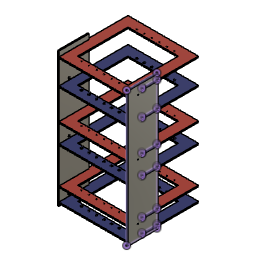
ionenantrieb v1 v3 (Autodesk Fusion 360 design; units mm, degrees)
Autodesk Fusion 360 part; units mm, degrees
sketch "Skizze1" plane through (0, 0, 0) normal (0, 0, 1) x (1, 0, 0)
  line L0 (0, 0) -> (100, 0)
  line L1 (100, 0) -> (100, 100)
  line L2 (100, 100) -> (0, 100)
  line L3 (0, 100) -> (0, 0)
  line L4 (-17.4, -20) -> (120, -20)
  line L5 (120, -20) -> (120, 120)
  line L6 (120, 120) -> (-20, 120)
  line L7 (-20, 120) -> (-20, 10)
  line L8 (-20, 10) -> (-17.4, 10)
  line L9 (-17.4, 10) -> (-17.4, -20)
  line L10 (50, 0) -> (50, 5)
  line L11 (117.4, 10) -> (117.4, -20)
  line L12 (120, 10) -> (117.4, 10)
  dimension "d1" = 100
  dimension "d2" = 100
  dimension "d4" = 2.6
  dimension "d5" = 30
  constraint horizontal L0
  constraint vertical L1
  constraint horizontal L2
  constraint vertical L3
  constraint coincident L0.start L3.end
  constraint perpendicular L7 L8
  constraint perpendicular L4 L9
  constraint parallel L0 L4
  constraint parallel L1 L5
  constraint parallel L2 L6
  constraint parallel L3 L7
  constraint midpoint L0 L10.start
  constraint perpendicular L0 L10
  constraint symmetric L7.end L10 L12.start
  constraint symmetric L8.end L10 L11.start
  constraint symmetric L4.start L10 L11.end
  measures "d1" distance of L1.end L2.end
  measures "d2" distance of L0.start L2.end
  measures "d4" distance of L7.end L8.end
  measures "d5" distance of L8.end L4.start
extrude "Extrusion1" add sketch "Skizze1" along normal blind 2.5 contours L4 L5 L6 L7 L8 L9 L11 L12 makes body 1
sketch "Skizze2" plane through (-17.4, 0, 0) normal (-1, 0, 0) x (0, -1, 0)
  line L0 (20, -5) -> (20, 117.8288)
  line L1 (-10, 0) -> (20, 0)
  line L2 (20, -5) -> (-40, -5)
  line L3 (-40, -5) -> (-40, -0.05)
  line L4 (-40, -0.05) -> (-10, -0.05)
  line L5 (-10, -0.05) -> (-10, 2.55)
  line L6 (-10, 2.55) -> (-40, 2.55)
  line L7 (-40, 2.55) -> (-40, 27.55)
  line L8 (-40, 15.05) -> (-27, 15.05)
  line L9 (-40, 30.15) -> (-10, 30.15)
  line L10 (-10, 30.15) -> (-10, 27.55)
  line L11 (-10, 27.55) -> (-40, 27.55)
  line L12 (-40, 30.15) -> (-40, 99.95)
  line L13 (-40, 102.55) -> (-10, 102.55)
  line L14 (-10, 102.55) -> (-10, 99.95)
  line L15 (-10, 199.95) -> (-40, 199.95)
  line L16 (-10, 202.55) -> (-10, 199.95)
  line L17 (-40, 202.55) -> (-10, 202.55)
  line L18 (-10, 138.4115) -> (-40, 138.4115)
  line L19 (-10, 141.0115) -> (-10, 138.4115)
  line L20 (-40, 141.0115) -> (-10, 141.0115)
  line L21 (-10, 249.95) -> (-40, 249.95)
  line L22 (-40, 252.55) -> (-10, 252.55)
  line L23 (-10, 252.55) -> (-10, 249.95)
  line L24 (-40, 252.55) -> (-40, 262.55)
  line L25 (-40, 262.55) -> (20, 262.55)
  line L26 (20, 262.55) -> (20, 117.8288)
  line L27 (-40, 249.95) -> (-40, 202.55)
  line L28 (-40, 199.95) -> (-40, 141.0115)
  line L29 (-40, 138.4115) -> (-40, 102.55)
  line L30 (-40, 99.95) -> (-10, 99.95)
  dimension "d37" = 5
  dimension "d38" = 4.95
  dimension "d39" = 2.6
  dimension "d40" = 25
  dimension "d41" = 100
  dimension "d42" = 10
  dimension "d43" = 60
  dimension "d44" = 60
  dimension "d45" = 60
  dimension "d46" = 60
  dimension "d47" = 60
  dimension "d49" = 60
  constraint vertical L0
  constraint perpendicular L0 L2
  constraint perpendicular L2 L3
  constraint perpendicular L3 L4
  constraint perpendicular L1 L5
  constraint perpendicular L5 L6
  constraint perpendicular L6 L7
  constraint midpoint L7 L8.start
  constraint perpendicular L7 L8
  constraint symmetric L3.end L8 L9.start
  constraint symmetric L4.end L8 L9.end
  constraint symmetric L5.end L8 L10.end
  constraint symmetric L6.end L8 L7.end
  constraint perpendicular L9 L12
  constraint perpendicular L22 L24
  constraint perpendicular L24 L25
  constraint perpendicular L17 L27
  constraint perpendicular L20 L28
  constraint perpendicular L13 L29
  constraint perpendicular L14 L30
  measures "d37" distance of L0.start L1
  measures "d38" distance of L2.end L3.end
  measures "d39" distance of L4.end L5.end
  measures "d40" distance of L6.end L7.end
  measures "d41" distance of L3.end L12.end
  measures "d42" distance of L22.start L24.end
  measures "d43" distance of L0.start L2.end
  measures "d44" distance of L0 L7
  measures "d45" distance of L0.end L29
  measures "d46" distance of L26 L28
  measures "d47" distance of L26 L27
  measures "d49" distance of L24 L26
extrude "Extrusion2" add sketch "Skizze2" along normal blind 2.5 separate body makes body 2
ref_plane "Arbeitsebene1" through (-18.65, 25, 15.05) normal (0, 0, 1) x (0, 1, 0)
mirror "Spiegeln1" about plane through (-18.65, 25, 15.05) normal (0, 0, 1) of bodies 1 makes body 3
ref_plane "Arbeitsebene2" through (50, 65, 28.85) normal (1, 0, 0) x (0, 1, 0)
mirror "Spiegeln2" about plane through (50, 65, 28.85) normal (1, 0, 0) of bodies 2 makes body 4
sketch "Skizze3" plane through (0, 0, 2.5) normal (0, 0, 1) x (-1, 0, 0)
  line L0 (0, 0) -> (0, -100)
  line L1 (0, -100) -> (-100, -100)
  line L2 (-100, -100) -> (-100, 0)
  line L3 (-100, 0) -> (0, 0)
  line L4 (-120, -120) -> (20, -120)
  line L5 (20, -120) -> (20, -10)
  line L6 (20, -10) -> (17.4, -10)
  line L7 (17.4, -10) -> (17.4, 20)
  line L8 (17.4, 20) -> (-117.4, 20)
  line L9 (-117.4, 20) -> (-117.4, -10)
  line L10 (-117.4, -10) -> (-120, -10)
  line L11 (-120, -10) -> (-120, -120)
  circle A0 centre (-12.5, -105) radius 2
  circle A1 centre (-27.5, -105) radius 2
  circle A2 centre (-42.5, -105) radius 2
  circle A3 centre (-57.5, -105) radius 2
  circle A4 centre (-72.5, -105) radius 2
  line L12 (0, -50) -> (-0.7928, -50)
  circle A5 centre (-27.5, 5) radius 2
  circle A6 centre (-72.5, 5) radius 2
  circle A7 centre (-42.5, 5) radius 2
  circle A8 centre (-57.5, 5) radius 2
  circle A9 centre (-12.5, 5) radius 2
  circle A10 centre (-87.5, -105) radius 2
  circle A11 centre (-87.5, 5) radius 2
  point P0 (-87.5, 5)
  dimension "d16" = 4
  dimension "d17" = 5
  dimension "d18" = 12.5
  dimension "d21" = 75
  dimension "d22" = 0
  constraint midpoint L0 L12.start
  constraint perpendicular L0 L12
  constraint symmetric A0 L12 A9
  constraint symmetric A1 L12 A5
  constraint symmetric A2 L12 A7
  constraint symmetric A3 L12 A8
  constraint symmetric A4 L12 A6
  constraint symmetric L12 A10.centre P0
  constraint symmetric L12 A10 A11
  measures "d16" diameter of A0
  measures "d17" distance of L1 A0.centre
  measures "d18" distance of L0 A0.centre
extrude "Extrusion3" cut sketch "Skizze3" against normal blind 2.5 contours A0 | A1 | A2 | A3 | A4 | A5 | A6 | A7 | A8 | A9 | A10 | A11 bodies 1
sketch "Skizze4" plane through (0, 0, 30.1) normal (0, 0, 1) x (-1, 0, 0)
  line L0 (0, 0) -> (0, -100)
  line L1 (0, -100) -> (-100, -100)
  line L2 (-100, -100) -> (-100, 0)
  line L3 (-100, 0) -> (0, 0)
  line L4 (-120, -120) -> (20, -120)
  line L5 (20, -120) -> (20, -10)
  line L6 (20, -10) -> (17.4, -10)
  line L7 (17.4, -10) -> (17.4, 20)
  line L8 (17.4, 20) -> (-117.4, 20)
  line L9 (-117.4, 20) -> (-117.4, -10)
  line L10 (-117.4, -10) -> (-120, -10)
  line L11 (-120, -10) -> (-120, -120)
  circle A0 centre (-12.5, -105) radius 1
  circle A1 centre (-27.5, -105) radius 1
  circle A2 centre (-42.5, -105) radius 1
  circle A3 centre (-57.5, -105) radius 1
  circle A4 centre (-72.5, -105) radius 1
  line L12 (0, -50) -> (-0.625, -50)
  circle A5 centre (-27.5, 5) radius 1
  circle A6 centre (-72.5, 5) radius 1
  circle A7 centre (-42.5, 5) radius 1
  circle A8 centre (-12.5, 5) radius 1
  circle A9 centre (-57.5, 5) radius 1
  circle A10 centre (-87.5, -105) radius 1
  circle A11 centre (-87.5, 5) radius 1
  dimension "d25" = 2
  dimension "d26" = 5
  dimension "d27" = 12.5
  dimension "d30" = 75
  dimension "d31" = 0
  constraint midpoint L0 L12.start
  constraint perpendicular L0 L12
  constraint symmetric A0 L12 A8
  constraint symmetric A1 L12 A5
  constraint symmetric A2 L12 A7
  constraint symmetric A3 L12 A9
  constraint symmetric A4 L12 A6
  constraint symmetric L12 A10 A11
  measures "d25" diameter of A0
  measures "d26" distance of L1 A0.centre
  measures "d27" distance of L0 A0.centre
extrude "Extrusion4" cut sketch "Skizze4" against normal blind 2.5 contours A0 | A1 | A2 | A3 | A4 | A5 | A6 | A7 | A8 | A9 | A10 | A11 bodies 3
sketch "Skizze5" plane through (117.4, 0, 0) normal (-1, 0, 0) x (0, -1, 0)
  line L0 (-40, 30.15) -> (-10, 30.15)
  line L1 (-10, 30.15) -> (-10, 27.55)
  line L2 (-10, 27.55) -> (-40, 27.55)
  line L3 (-40, 27.55) -> (-40, 2.55)
  line L4 (-40, 2.55) -> (-10, 2.55)
  line L5 (-10, 2.55) -> (-10, -0.05)
  line L6 (-10, -0.05) -> (-40, -0.05)
  line L7 (-40, -0.05) -> (-40, -5)
  line L8 (-40, -5) -> (20, -5)
  line L9 (20, -5) -> (20, 262.55)
  line L10 (20, 262.55) -> (-40, 262.55)
  line L11 (-40, 262.55) -> (-40, 252.55)
  line L12 (-40, 252.55) -> (-10, 252.55)
  line L13 (-10, 252.55) -> (-10, 249.95)
  line L14 (-10, 249.95) -> (-40, 249.95)
  line L15 (-40, 249.95) -> (-40, 202.55)
  line L16 (-40, 202.55) -> (-10, 202.55)
  line L17 (-10, 202.55) -> (-10, 199.95)
  line L18 (-10, 199.95) -> (-40, 199.95)
  line L19 (-40, 199.95) -> (-40, 141.0115)
  line L20 (-40, 141.0115) -> (-10, 141.0115)
  line L21 (-10, 141.0115) -> (-10, 138.4115)
  line L22 (-10, 138.4115) -> (-40, 138.4115)
  line L23 (-40, 138.4115) -> (-40, 102.55)
  line L24 (-40, 102.55) -> (-10, 102.55)
  line L25 (-10, 102.55) -> (-10, 99.95)
  line L26 (-10, 99.95) -> (-40, 99.95)
  line L27 (-40, 99.95) -> (-40, 30.15)
sketch "Skizze6" plane through (-19.9, 0, 0) normal (-1, 0, 0) x (0, -1, 0)
  line L0 (-40, 30.15) -> (-10, 30.15)
  line L1 (-10, 30.15) -> (-10, 27.55)
  line L2 (-10, 27.55) -> (-40, 27.55)
  line L3 (-40, 27.55) -> (-40, 2.55)
  line L4 (-40, 2.55) -> (-10, 2.55)
  line L5 (-10, 2.55) -> (-10, -0.05)
  line L6 (-10, -0.05) -> (-40, -0.05)
  line L7 (-40, -0.05) -> (-40, -5)
  line L8 (-40, -5) -> (20, -5)
  line L9 (20, -5) -> (20, 262.55)
  line L10 (20, 262.55) -> (-40, 262.55)
  line L11 (-40, 262.55) -> (-40, 252.55)
  line L12 (-40, 252.55) -> (-10, 252.55)
  line L13 (-10, 252.55) -> (-10, 249.95)
  line L14 (-10, 249.95) -> (-40, 249.95)
  line L15 (-40, 249.95) -> (-40, 202.55)
  line L16 (-40, 202.55) -> (-10, 202.55)
  line L17 (-10, 202.55) -> (-10, 199.95)
  line L18 (-10, 199.95) -> (-40, 199.95)
  line L19 (-40, 199.95) -> (-40, 141.0115)
  line L20 (-40, 141.0115) -> (-10, 141.0115)
  line L21 (-10, 141.0115) -> (-10, 138.4115)
  line L22 (-10, 138.4115) -> (-40, 138.4115)
  line L23 (-40, 138.4115) -> (-40, 102.55)
  line L24 (-40, 102.55) -> (-10, 102.55)
  line L25 (-10, 102.55) -> (-10, 99.95)
  line L26 (-10, 99.95) -> (-40, 99.95)
  line L27 (-40, 99.95) -> (-40, 30.15)
  circle A0 centre (0, 6.55) radius 2
  circle A1 centre (0, 106.55) radius 2
  circle A2 centre (0, 206.55) radius 2
  dimension "d50" = 4
  dimension "d51" = 4
  dimension "d52" = 4
  dimension "d53" = 4
  dimension "d54" = 4
  dimension "d55" = 4
  measures "d50" diameter of A0
  measures "d51" distance of L4 A0.centre
  measures "d52" diameter of A2
  measures "d53" diameter of A1
  measures "d54" distance of L24 A1.centre
  measures "d55" distance of L16 A2.centre
extrude "Extrusion5" cut sketch "Skizze6" against normal blind 2.5 contours A0 | A1 | A2 bodies 2
copy_body "Körper->Berechn1" bodies 1 removing the originals makes body 5 in component "Component"
copy_body "Körper->Berechn2" bodies 3 removing the originals makes body 6 in component "Component'"
copy_body "Körper->Berechn3" bodies 4 removing the originals makes body 7 in component "Component''"
copy_body "Körper->Berechn4" bodies 2 removing the originals makes body 8 in component "Component'''"
copy_body "Körper kopieren/einfügen1" bodies 6 makes body 9
move_body "Verschieben2" bodies 9 to x (1, 0, 0) y (0, 1, 0) z (0, 0, 1) at (0, 0, 70)
copy_body "Körper->Berechn5" bodies 9 removing the originals makes body 10 in component "Component''''"
move_body "Verschieben1" bodies 10 to x (1, 0, 0) y (0, 1, 0) z (0, 0, 1) at (0, 0, -0.05) in component "Component''''"
copy_body "Körper kopieren/einfügen2" bodies 5 makes body 11
move_body "Verschieben3" bodies 11 to x (1, 0, 0) y (0, 1, 0) z (0, 0, 1) at (0, 0, 60)
copy_body "Körper->Berechn6" bodies 11 removing the originals makes body 12 in component "Component'''''"
move_body "Verschieben1'" bodies 12 to x (1, 0, 0) y (0, 1, 0) z (0, 0, 1) at (0, 0, 40) in component "Component'''''"
copy_body "Körper kopieren/einfügen3" bodies 10 makes body 13
move_body "Verschieben4" bodies 13 to x (1, 0, 0) y (0, 1, 0) z (0, 0, 1) at (0, 0, 152.45)
copy_body "Körper kopieren/einfügen4" bodies 12 makes body 14
move_body "Verschieben5" bodies 14 to x (1, 0, 0) y (0, 1, 0) z (0, 0, 1) at (0, -0.05, 100.05)
sketch "Skizze7" plane through (119.9, 0, 0) normal (1, 0, 0) x (0, 1, 0)
  line L0 (10, 30.15) -> (40, 30.15)
  line L1 (40, 30.15) -> (40, 99.95)
  line L2 (40, 99.95) -> (10, 99.95)
  line L3 (10, 99.95) -> (10, 102.55)
  line L4 (10, 102.55) -> (40, 102.55)
  line L5 (40, 102.55) -> (40, 138.4115)
  line L6 (40, 138.4115) -> (10, 138.4115)
  line L7 (10, 138.4115) -> (10, 141.0115)
  line L8 (10, 141.0115) -> (40, 141.0115)
  line L9 (40, 141.0115) -> (40, 199.95)
  line L10 (40, 199.95) -> (10, 199.95)
  line L11 (10, 199.95) -> (10, 202.55)
  line L12 (10, 202.55) -> (40, 202.55)
  line L13 (40, 202.55) -> (40, 249.95)
  line L14 (40, 249.95) -> (10, 249.95)
  line L15 (10, 249.95) -> (10, 252.55)
  line L16 (10, 252.55) -> (40, 252.55)
  line L17 (40, 252.55) -> (40, 262.55)
  line L18 (40, 262.55) -> (-20, 262.55)
  line L19 (-20, 262.55) -> (-20, -5)
  line L20 (-20, -5) -> (40, -5)
  line L21 (40, -5) -> (40, -0.05)
  line L22 (40, -0.05) -> (10, -0.05)
  line L23 (10, -0.05) -> (10, 2.55)
  line L24 (10, 2.55) -> (40, 2.55)
  line L25 (40, 2.55) -> (40, 27.55)
  line L26 (40, 27.55) -> (10, 27.55)
  line L27 (10, 27.55) -> (10, 30.15)
  circle A0 centre (0, 245.95) radius 1
  circle A1 centre (0, 23.55) radius 1
  circle A2 centre (0, 134.4115) radius 1
  dimension "d58" = 2
  dimension "d60" = 2
  dimension "d61" = 4
  dimension "d62" = 2
  dimension "d64" = 4
  dimension "d65" = 4
  measures "d58" diameter of A0
  measures "d60" diameter of A1
  measures "d61" distance of L26 A1.centre
  measures "d62" diameter of A2
  measures "d64" distance of L14 A0.centre
  measures "d65" distance of L6 A2.centre
extrude "Extrusion1'" cut sketch "Skizze7" against normal blind 2.5 contours A0 | A1 | A2 bodies 7 in component "Component''"
component "Component" placed x (1, 0, 0) y (0, 1, 0) z (0, 0, 1) at (0, 0, 0)
component "Component'" placed x (1, 0, 0) y (0, 1, 0) z (0, 0, 1) at (0, 0, 0)
component "Component''" placed x (1, 0, 0) y (0, 1, 0) z (0, 0, 1) at (0, 0, 0)
component "Component'''" placed x (1, 0, 0) y (0, 1, 0) z (0, 0, 1) at (0, 0, 0)
component "Component''''" placed x (1, 0, 0) y (0, 1, 0) z (0, 0, 1) at (0, 0, 40.9115)
component "Component'''''" placed x (1, 0, 0) y (0, 1, 0) z (0, 0, 1) at (0, 0, 0)
component "Component''''''" placed x (1, 0, 0) y (0, 1, 0) z (0, 0, 1) at (0, 0, 0)
equation "d18 = ( 100 / 8 ) * 1 mm"
equation "d21 = 100 mm - ( 2 * 100 / 8 ) * 1 mm"
equation "d27 = ( 100 / 8 ) * 1 mm"
equation "d30 = 100 mm - ( 2 * 100 / 8 ) * 1 mm"
